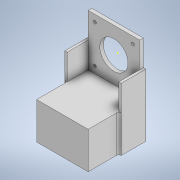
# Autodesk Inventor part: Motor mount
Saved by Autodesk Inventor 2020 (Build 240168000, 168)
## iProperties
Created: 2021-06-19
Part Number: Motor mount
Material: Generic
Document SubType Name: Modeling
Designer: ugwue
Density: 1 g/cm^3
Appearance: Default
Author: ugwue
Autodesk Inventor part; units mm, degrees
ref_plane "YZ Plane" through (0, 0, 0) normal (1, 0, 0) x (0, 1, 0)
ref_plane "XZ Plane" through (0, 0, 0) normal (0, 1, 0) x (-1, 0, 0)
ref_plane "XY Plane" through (0, 0, 0) normal (0, 0, 1) x (1, 0, 0)
sketch "Sketch1" plane through (0, 0, 0) normal (0, 0, 1) x (1, 0, 0)
  circle A0 centre (0, 0) radius 11.5
  line L0 (-21, 21) -> (21, 21)
  line L1 (21, 21) -> (21, -21)
  line L2 (-21, -21) -> (-21, 21)
  line L3 (-21, 21) -> (21, -21) construction
  line L4 (21, 21) -> (-21, -21) construction
  line L5 (21, -21) -> (21, -51)
  line L6 (21, -51) -> (-21, -51)
  line L7 (-21, -51) -> (-21, -21)
  dimension "d0" = 23
  constraints: 16 end point, 2 midpoint, 2 parallel, 1 centre point, 1 coincident, 1 horizontal, 1 perpendicular
  measures "d0" diameter of A0
extrude "Extrusion1" add sketch "Sketch1" along normal blind 3
sketch "Sketch2" plane through (0, 0, 3) normal (0, 0, 1) x (1, 0, 0)
  line L0 (-15.5, -15.5) -> (15.5, 15.5) construction
  line L1 (15.5, -15.5) -> (-15.5, 15.5) construction
  circle A0 centre (-15.5, 15.5) radius 1.25
  circle A1 centre (15.5, 15.5) radius 1.25
  circle A2 centre (15.5, -15.5) radius 1.25
  circle A3 centre (-15.5, -15.5) radius 1.25
  point P0 (0, 0)
  dimension "d6" = 31
  dimension "d7" = 31
  dimension "d8" = 2.5
  dimension "d9" = 2.5
  dimension "d10" = 2.5
  dimension "d11" = 2.5
  constraints: 4 centre point, 4 end point, 3 coincident, 2 midpoint
  measures "d6" distance of L0.start L1.start
  measures "d7" distance of L0.end L1.start
  measures "d8" diameter of A0
  measures "d9" diameter of A1
  measures "d10" diameter of A2
  measures "d11" diameter of A3
extrude "Extrusion2" cut sketch "Sketch2" against normal blind 3
sketch "Sketch3" plane through (0, 0, 3) normal (0, 0, 1) x (1, 0, 0)
  line L0 (-21, 21) -> (21, 21)
  line L1 (21, -21) -> (-21, -21)
  line L2 (-21, -51) -> (21, -51)
  line L3 (21, -51) -> (21, -21)
  line L4 (21, -21) -> (-21, -21)
  line L5 (-21, -21) -> (-21, -51)
  point P0 (0, 0)
  constraints: 12 end point, 3 parallel, 2 horizontal, 1 perpendicular
extrude "Extrusion3" add sketch "Sketch3" along normal blind 42
sketch "Sketch4" plane through (0, 0, 0) normal (0, 0, -1) x (-1, 0, 0)
  line L0 (-21, -51) -> (-21, 21) projected
  line L1 (-21, -51) -> (-23, -51)
  line L2 (-23, -51) -> (-23, 0)
  line L3 (-23, 0) -> (-21, 0)
  line L4 (-21, 0) -> (-21, -51)
  line L5 (21, -51) -> (-21, -51) projected
  line L6 (21, -51) -> (23, -51)
  line L7 (23, -51) -> (23, 0)
  line L8 (23, 0) -> (21, 0)
  line L9 (21, 0) -> (21, -51)
  point P0 (0, 0)
  dimension "d17" = 2
  dimension "d18" = 2
  dimension "d19" = 51
  constraints: 16 end point, 4 parallel, 2 horizontal, 2 perpendicular
  measures "d17" distance of L2.end L3.end
  measures "d18" distance of L8.end L7.end
  measures "d19" distance of L7.end L6.end
extrude "Extrusion4" add sketch "Sketch4" against normal blind 20
sketch "Sketch5" plane through (-21, -51, 45) normal (0, -1, 0) x (1, 0, 0)
  line L0 (42, -42) -> (0, -42) projected
  line L1 (39, -3) -> (2.4954, -3)
  line L2 (2.4954, -3) -> (2.4954, -42)
  line L3 (2.4954, -42) -> (39, -42)
  line L4 (39, -42) -> (39, -3)
  point P0 (21, -45)
  constraints: 8 end point, 2 parallel, 1 horizontal, 1 perpendicular, 1 point on line
extrude "Extrusion5" cut sketch "Sketch5" against normal blind 25
fillet "Fillet1" radius 2 2 edges at (-21, -36, 20) (21, -36, 20)
sketch "Sketch6" plane through (0, 0, 0) normal (0, 0, -1) x (-1, 0, 0)
  point P0 (0, 0)
body "Solid1"
